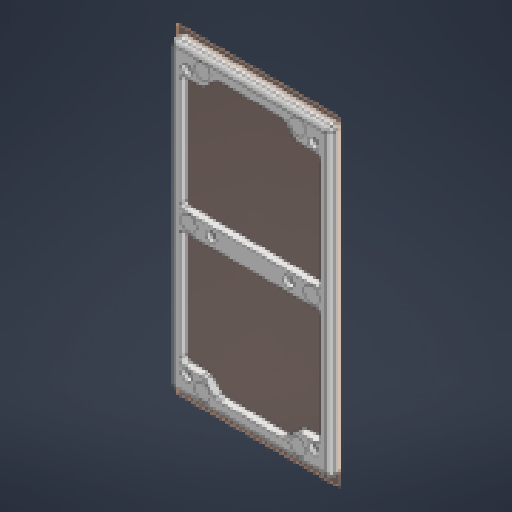
# Autodesk Inventor part: BP_ShroudAdapter
Saved by Autodesk Inventor 2026.1 (Build 301233020, 233B)
## iProperties
Created: 2025-09-13
Part Number: BP_ShroudAdapter
Material: Generic
Document SubType Name: Modeling
Designer: atrus
Density: 1 g/cm^3
Appearance: Default
Author: atrus
Autodesk Inventor part; units mm, degrees
ref_plane "YZ Plane" through (0, 0, 0) normal (1, 0, 0) x (0, 1, 0)
ref_plane "XZ Plane" through (0, 0, 0) normal (0, 1, 0) x (-1, 0, 0)
ref_plane "XY Plane" through (0, 0, 0) normal (0, 0, 1) x (1, 0, 0)
ref_plane "Work Plane1" through (0, 0, 0) normal (0, 0, 1) x (1, 0, 0)
sketch "Sketch1" plane through (0, 0, 0) normal (0, 0, 1) x (1, 0, 0)
  line L0 (49.666, 21.9) -> (49.666, 96.1) projected
  line L1 (-49.666, 96.1) -> (-49.666, 21.9) projected
  line L2 (-49.666, -96.1) -> (49.666, -96.1) projected
  line L3 (-49.666, -21.9) -> (-49.666, -96.1) projected
  line L4 (49.666, -21.9) -> (49.666, -96.1) projected
  line L5 (49.666, -21.9) -> (49.666, 21.9)
  line L6 (-49.666, 21.9) -> (-49.666, -21.9)
  line L7 (-51.666, -98.1) -> (51.666, -98.1)
  line L8 (51.666, -98.1) -> (51.666, -21.9)
  line L9 (51.666, -21.9) -> (51.666, 21.9)
  line L10 (51.666, 21.9) -> (51.666, 98.1)
  line L11 (51.666, 98.1) -> (-51.666, 98.1)
  line L12 (-51.666, 98.1) -> (-51.666, 21.9)
  line L13 (-51.666, 21.9) -> (-51.666, -21.9)
  line L14 (-51.666, -21.9) -> (-51.666, -98.1)
  line L15 (-45.666, 21.9) -> (-45.666, 92.1)
  line L16 (-45.666, 92.1) -> (45.666, 92.1)
  line L17 (45.666, 92.1) -> (45.666, 21.9)
  line L18 (45.666, 21.9) -> (45.666, -21.9)
  line L19 (45.666, -21.9) -> (45.666, -92.1)
  line L20 (45.666, -92.1) -> (-45.666, -92.1)
  line L21 (-45.666, -92.1) -> (-45.666, -21.9)
  line L22 (-45.666, -21.9) -> (-45.666, 21.9)
  line L23 (49.666, 96.1) -> (-49.666, 96.1) projected
  point P0 (0, 0)
  dimension "d0" = 2
  dimension "d1" = 4
  dimension "d41" = 2
  dimension "d42" = 4
  dimension "d43" = 2
  constraints: 36 end point, 3 parallel, 1 vertical, 10 other
  measures "d0" distance between parallel lines of L14 L3
  measures "d1" distance between parallel lines of L1 L15
  measures "d41" distance between parallel lines of L23 L11
  measures "d42" distance between parallel lines of L23 L16
  measures "d43" distance between parallel lines of L10 L0
extrude "Extrusion1" add sketch "Sketch1" along normal blind 5 contours L5 L4 L2 L3 L6 L1 L23 L0 | L14 L13 L12 L11 L10 L9 L8 L7
sketch "Sketch2" plane through (0, 0, 0) normal (0, 0, -1) x (-1, 0, 0)
  line L0 (-51.666, 98.1) -> (51.666, 98.1) projected
  line L1 (-51.666, 98.1) -> (51.666, 98.1)
  line L2 (51.666, 98.1) -> (51.666, -98.1)
  line L3 (51.666, -98.1) -> (-51.666, -98.1)
  line L4 (-51.666, -98.1) -> (-51.666, 98.1)
  line L5 (49.866, -96.3) -> (-49.866, -96.3)
  line L6 (-49.866, -96.3) -> (-49.866, 96.3)
  line L7 (-49.866, 96.3) -> (49.866, 96.3)
  line L8 (49.866, 96.3) -> (49.866, -96.3)
  point P0 (0, 0)
  dimension "d4" = 1.8
  dimension "d5" = 1.8
  dimension "d6" = 1.8
  dimension "d7" = 1.8
  constraints: 16 end point, 4 parallel, 2 horizontal, 2 perpendicular
  measures "d4" distance between parallel lines of L0 L7
  measures "d5" distance between parallel lines of L4 L6
  measures "d6" distance between parallel lines of L2 L8
  measures "d7" distance between parallel lines of L3 L5
extrude "Extrusion2" add sketch "Sketch2" along normal blind 2.8
sketch "Sketch3" plane through (0, 0, 5) normal (0, 0, 1) x (1, 0, 0)
  line L0 (-45.666, -92.1) -> (-45.666, 92.1) projected
  line L1 (45.666, 92.1) -> (45.666, -92.1) projected
  line L2 (-45.666, -6) -> (45.666, -6)
  line L3 (45.666, -6) -> (45.666, 6)
  line L4 (45.666, 6) -> (-45.666, 6)
  line L5 (-45.666, 6) -> (-45.666, -6)
  line L6 (-37.45, -82) -> (-37.45, -89) projected
  line L7 (-37.45, -92.1) -> (-45.666, -92.1)
  line L8 (37.45, -82) -> (37.45, -89) projected
  line L9 (-37.45, 89.1) -> (-37.45, 82.1) projected
  line L10 (37.45, 82.1) -> (37.45, 89.1) projected
  line L11 (45.666, -92.1) -> (-45.666, -92.1) projected
  line L12 (45.666, -92.1) -> (37.45, -92.1)
  line L13 (45.666, 92.1) -> (45.666, -92.1) projected
  line L14 (45.666, -92.1) -> (45.666, -82)
  line L15 (-45.666, 92.1) -> (45.666, 92.1) projected
  line L16 (37.45, 92.309) -> (45.666, 92.1)
  line L17 (45.666, 92.1) -> (45.666, 82.1)
  line L18 (-37.45, 89.1) -> (-37.45, 92.1)
  line L19 (-45.666, 92.1) -> (45.666, 92.1) projected
  line L20 (45.666, 81.1) -> (-45.666, 81.1)
  line L21 (45.666, -81.1) -> (-45.666, -81.1)
  point P0 (0, 0)
  point P1 (45.666, 0)
  point P2 (45.666, -6)
  dimension "d10" = 12
  dimension "d21" = 11
  dimension "d22" = 11
  constraints: 24 end point, 10 point on line, 4 perpendicular, 2 midpoint, 2 parallel, 1 horizontal
  measures "d10" distance between parallel lines of L2 L4
  measures "d21" distance between parallel lines of L15 L20
  measures "d22" distance between parallel lines of L11 L21
extrude "Extrusion3" add sketch "Sketch3" against normal blind 5 contours L0 L21 L1 L11 L7 | L0 L4 L1 L2 | L0 L15 L1 L20
sketch "Sketch4" plane through (0, 0, 5) normal (0, 0, 1) x (1, 0, 0)
  circle A0 centre (-25, 0) radius 1.9 construction
  circle A1 centre (25, 0) radius 1.9 construction
  circle A2 centre (-40.95, -85.5) radius 1.9 construction
  circle A3 centre (40.95, -85.5) radius 1.9 construction
  circle A4 centre (-40.95, 85.6) radius 1.9 construction
  circle A5 centre (40.95, 85.6) radius 1.9 construction
  point P0 (0, 0)
  constraints: 6 coincident
hole "Hole1" at (-25, 0, 5) at (25, 0, 5) at (-40.95, 85.6, 5) at (40.95, 85.6, 5) at (40.95, -85.5, 5) at (-40.95, -85.5, 5) direction (0, 0, -1) diameter 3.4 end through all counterbore diameter 6.5 counterbore depth 3 clearance for "Socket Head Cap Screw" size "M3" standard "Ansi Metric M Profile"
fillet "Fillet1" radius 2 8 edges at (51.666, 98.1, 1.1) (-51.666, 98.1, 1.1) (51.666, -98.1, 1.1) (-51.666, -98.1, 1.1) (-45.666, 6, 2.5) (45.666, 6, 2.5) (45.666, -6, 2.5) (-45.666, -6, 2.5)
sketch "Sketch5" plane through (0, 0, 5) normal (0, 0, 1) x (1, 0, 0)
  circle A0 centre (30.666, 89.6) radius 5.1
  circle A1 centre (-30.666, 89.6) radius 5.1
  circle A2 centre (39.666, 0) radius 5.1
  circle A3 centre (-39.666, 0) radius 5.1
  circle A4 centre (30.666, -89.6) radius 5.1
  circle A5 centre (-30.666, -89.6) radius 5.1
  line L0 (-45.666, -81.1) -> (45.666, -81.1) projected
  line L1 (0, -81.1) -> (0, -98.1) construction
  line L2 (-49.666, -98.1) -> (49.666, -98.1) projected
  line L3 (0, -89.6) -> (-51.666, -89.6) construction
  line L4 (-51.666, 96.1) -> (-51.666, -96.1) projected
  line L5 (0, -89.6) -> (51.666, -89.6) construction
  line L6 (51.666, -96.1) -> (51.666, 96.1) construction
  line L7 (51.666, 0) -> (-51.666, 0) construction
  line L8 (45.666, 81.1) -> (-45.666, 81.1) construction
  line L9 (0, 81.1) -> (0, 98.1) construction
  line L10 (-49.666, 98.1) -> (49.666, 98.1) construction
  line L11 (0, 89.6) -> (-51.666, 89.6) construction
  line L12 (0, 89.6) -> (51.666, 89.6) construction
  point P0 (0, 0)
  dimension "d23" = 10.2
  dimension "d24" = 21
  dimension "d25" = 21
  dimension "d26" = 12
  dimension "d27" = 12
  constraints: 14 end point, 12 point on line, 8 midpoint, 6 centre point, 5 equal radius, 2 horizontal, 2 vertical alignment, 1 perpendicular
  measures "d23" diameter of A4
  measures "d24" distance of L5.end A4.centre
  measures "d25" distance from line of L4 A5.centre
  measures "d26" distance of L7.end A3.centre
  measures "d27" distance of L7.start A2.centre
extrude "Extrusion4" cut sketch "Sketch5" against normal blind 3.6
sketch "Sketch6" plane through (0, 0, 5) normal (0, 0, 1) x (1, 0, 0)
  circle A0 centre (30.666, 89.6) radius 5.1 projected
  circle A1 centre (-30.666, 89.6) radius 5.1 projected
  circle A2 centre (39.666, 0) radius 5.1 projected
  circle A3 centre (-39.666, 0) radius 5.1 projected
  circle A4 centre (30.666, -89.6) radius 5.1 projected
  circle A5 centre (-30.666, -89.6) radius 5.1 projected
  point P0 (0, 0)
extrude "Extrusion5" add sketch "Sketch6" against normal blind 0.2
fillet "Fillet2" radius 3 8 edges at (-51.0802, 97.5142, 5) (-51.666, 0, 5) (-51.0802, -97.5142, 5) (0, -98.1, 5) (51.0802, -97.5142, 5) (51.666, 0, 5) (51.0802, 97.5142, 5) (0, 98.1, 5)
sketch "Sketch7" plane through (0, 0, 5) normal (0, 0, 1) x (1, 0, 0)
  circle A0 centre (-30.666, -89.6) radius 5.1 construction
  circle A1 centre (30.666, -89.6) radius 5.1 construction
  circle A2 centre (-30.666, 89.6) radius 5.1 construction
  circle A3 centre (30.666, 89.6) radius 5.1 construction
  line L0 (45.666, -81.1) -> (-45.666, -81.1) construction
  line L1 (30.166, -81.1) -> (21.666, -89.6)
  line L2 (21.666, -89.6) -> (-21.666, -89.6)
  line L3 (-21.666, -89.6) -> (-30.166, -81.1)
  line L4 (48.666, 95.1) -> (48.666, -95.1) construction
  line L5 (48.666, 0) -> (-48.666, 0) construction
  line L6 (-48.666, -95.1) -> (-48.666, 95.1) construction
  line L7 (-30.166, -81.1) -> (30.166, -81.1)
  line L8 (30.166, 81.1) -> (21.666, 89.6)
  line L9 (21.666, 89.6) -> (-21.666, 89.6)
  line L10 (-21.666, 89.6) -> (-30.166, 81.1)
  line L11 (-30.166, 81.1) -> (30.166, 81.1)
  point P0 (0, 0)
  dimension "d35" = 135
  dimension "d36" = 9
  dimension "d37" = 9
  constraints: 18 end point, 4 symmetric about line, 2 midpoint, 2 point on line, 1 collinear, 1 horizontal alignment, 1 parallel, 1 perpendicular
  measures "d35" angle of L3 L2
  measures "d36" distance of A0.centre L2.end
  measures "d37" distance of A1.centre L1.end
extrude "Extrusion6" cut sketch "Sketch7" against normal blind 5
fillet "Fillet3" radius 3 12 edges at (-30.166, -81.1, 2.5) (-45.666, -81.1, 2.5) (-21.666, -89.6, 2.5) (21.666, -89.6, 2.5) (30.166, -81.1, 2.5) (45.666, -81.1, 2.5) (45.666, 81.1, 2.5) (30.166, 81.1, 2.5) (21.666, 89.6, 2.5) (-21.666, 89.6, 2.5) (-30.166, 81.1, 2.5) (-45.666, 81.1, 2.5)
body "Solid1"
